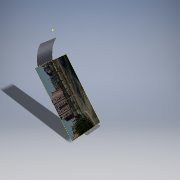
# Autodesk Inventor part: baraca
Saved by Autodesk Inventor 2019 (Build 230136000, 136)
## iProperties
Created: 2019-02-25
Part Number: baraca
Material: Generic
Document SubType Name: Modeling
Designer: gaincarlo
Density: 1 g/cm^3
Appearance: Slate - Random Gray
Author: gaincarlo
Autodesk Inventor part; units mm, degrees
ref_plane "YZ Plane" through (0, 0, 0) normal (1, 0, 0) x (0, 1, 0)
ref_plane "XZ Plane" through (0, 0, 0) normal (0, 1, 0) x (-1, 0, 0)
ref_plane "Work Plane2" through (0, 0, 10) normal (0, 0, 1) x (1, 0, 0)
sketch "Sketch3" plane through (0, 0, 10) normal (0, 0, 1) x (1, 0, 0)
  ellipse E0 centre (17474, -6711) end of major axis (949, -6904) minor radius 13089.7498 (3411.3173, 103.156) -> (19430.2058, -19700.5351) ccw
  line L0 (19491, -21143) -> (18773, -4107) construction
  line L1 (18773, -4107) -> (949, 778) construction
  line L2 (19430.2058, -19700.5351) -> (19428.267, -19680.9077)
  line L3 (3426.8947, 91.0588) -> (3411.3173, 103.156)
  spline S0 degree 5 poles (3426.8946, 91.0588) (3289.3305, -86.0799) (3155.5628, -266.1669) (3025.7448, -449.1474) (2582.6919, -1104.0004) (2192.609, -1792.9681) (1942.9072, -2302.662) (1514.5607, -3335.0424) (1219.6209, -4412.9944) (1108.6438, -4952.5138) (958.6777, -6038.7686) (952.3967, -7135.2681) (985.4333, -7680.7934) (1124.2205, -8773.4072) (1403.7291, -9838.831) (1579.2157, -10366.0927) (2003.0073, -11414.8396) (2552.3715, -12403.7993) (2862.1011, -12889.7087) (3552.2085, -13845.9501) (4345.5597, -14718.6835) (4775.5864, -15142.4306) (5700.1065, -15962.859) (6703.5469, -16684.8881) (7235.0599, -17028.5381) (8351.5895, -17677.3566) (9523.7658, -18219.4788) (10133.8388, -18468.5046) (11392.1439, -18918.5596) (12684.8119, -19257.7929) (13347.2554, -19401.6344) (14691.7872, -19635.0677) (16051.0972, -19755.979) (16737.5023, -19788.5174) (17688.8854, -19794.4714) (18638.3769, -19746.2443) (18902.0275, -19728.6554) (19165.3544, -19706.8781) (19428.267, -19680.9077) knots 0 0 0 0 0 0 0.034325 0.034325 0.034325 0.120975 0.120975 0.120975 0.205036 0.205036 0.205036 0.288433 0.288433 0.288433 0.373249 0.373249 0.373249 0.461235 0.461235 0.461235 0.553458 0.553458 0.553458 0.650175 0.650175 0.650175 0.75089 0.75089 0.75089 0.854514 0.854514 0.854514 0.959566 0.959566 0.959566 1 1 1 1 1 1
  point P0 (0, 0)
  dimension "d6" = 19.7229
  constraints: 8 end point, 2 point on line, 7 other
extrude "Extrusion3" add sketch "Sketch3" along normal blind 5000
ref_plane "Work Plane1" through (19428.267, -19680.9077, 5010) normal (0.7773315, 0.6290912, 0) x (0, 0, -1)
sketch "Sketch4" plane through (19428.267, -19680.9077, 5010) normal (0.7773315, 0.6290912, 0) x (0, 0, -1)
  line L0 (-4491.9999, 841.2222) -> (-4491.9999, 20653.222) construction
  line L1 (-4491.9999, 20653.222) -> (5414, 20653.222) construction
  line L2 (5414, 20653.222) -> (5414, 841.2222) construction
  line L3 (5414, 841.2222) -> (-4491.9999, 841.2222) construction
  point P0 (5010, 27520.7414)
  constraints: 2 other
body "Solid1"
